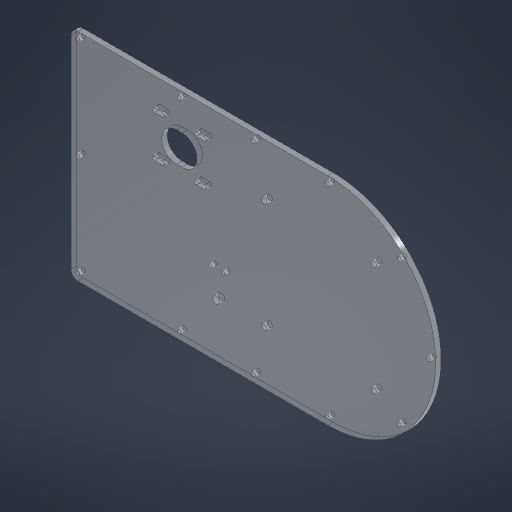
# Autodesk Inventor part: Base_solida
Saved by Autodesk Inventor 2025.2 (Build 292293000, 293)
## iProperties
Created: 2025-04-27
Part Number: Base_solida
Material: Acrilico
Document SubType Name: Modeling
Designer: Tiago
Density: 1.18 g/cm^3
Appearance: Polycarbonate - Clear
Mass: 159.889 g
Surface Area: 836.081 cm^2
Volume: 159.889 cm^3
Author: Tiago
Autodesk Inventor part; units mm, degrees
ref_plane "YZ Plane" through (0, 0, 0) normal (1, 0, 0) x (0, 1, 0)
ref_plane "XZ Plane" through (0, 0, 0) normal (0, 1, 0) x (-1, 0, 0)
ref_plane "XY Plane" through (0, 0, 0) normal (0, 0, 1) x (1, 0, 0)
sketch "Sketch1" plane through (0, 0, 0) normal (0, 0, 1) x (1, 0, 0)
  line L0 (-150, -80) -> (40, -80)
  line L1 (40, 80) -> (-150, 80)
  line L2 (-150, 80) -> (-150, -80)
  line L3 (-150, 0) -> (-107, 0) construction
  line L4 (-107, 0) -> (33.79, 0) construction
  line L5 (33.79, -40.6) -> (33.79, 40.6) construction
  line L6 (-6.81, 0) -> (74.39, 0) construction
  line L7 (33.79, 40.6) -> (74.39, 40.6) construction
  line L8 (74.39, 40.6) -> (74.39, 0) construction
  circle A0 centre (74.39, 40.6) radius 2
  circle A1 centre (74.39, -40.6) radius 2
  circle A2 centre (-6.81, 40.6) radius 2
  circle A3 centre (-6.81, -40.6) radius 2
  line L9 (33.79, 0) -> (33.79, 47) construction
  line L10 (33.79, 0) -> (33.79, -47) construction
  line L11 (150, 0) -> (120, 0) construction
  line L12 (120, 0) -> (120, 0)
  arc A4 (40, -80) -> (120, 0) centre (40, 0) ccw
  arc A5 (120, 0) -> (40, 80) centre (40, 0) ccw
  line L13 (120, 0) -> (115, 0) construction
  circle A6 centre (115, 0) radius 1.5
  line L14 (40, 0) -> (96.5685, 56.5685) construction
  line L15 (96.5685, -56.5685) -> (93.033, -53.033) construction
  circle A7 centre (93.033, -53.033) radius 1.5
  line L16 (40, -80) -> (40, -75) construction
  circle A8 centre (40, -75) radius 1.5
  line L17 (40, -75) -> (-15, -75) construction
  line L18 (-15, -75) -> (-70, -75) construction
  line L19 (-150, -75) -> (-145, -75) construction
  circle A9 centre (-15, -75) radius 1.5
  circle A10 centre (-70, -75) radius 1.5
  circle A11 centre (-145, -75) radius 1.5
  circle A12 centre (-145, 0) radius 1.5
  circle A13 centre (93.033, 53.033) radius 1.5
  circle A14 centre (40, 75) radius 1.5
  circle A15 centre (-15, 75) radius 1.5
  circle A16 centre (-70, 75) radius 1.5
  circle A17 centre (-145, 75) radius 1.5
  line L20 (-145, -80) -> (-145, -75) construction
  line L21 (-150, 0) -> (-145, 0) construction
  line L22 (-71.7142, 42.5) -> (-67.7142, 42.5) construction
  line L23 (33.79, 0) -> (31.29, 0) construction
  line L24 (33.79, 0) -> (45.79, 0) construction
  line L25 (45.79, 0) -> (45.79, 58) construction
  circle A18 centre (45.79, 58) radius 1.1
  circle A19 centre (45.79, 65) radius 1.1
  arc A20 (-82.2142, 56.5) -> (-82.2142, 59.5) centre (-82.2142, 58) ccw
  line L26 (-82.2142, 56.5) -> (-88.2142, 56.5)
  line L27 (-82.2142, 59.5) -> (-88.2142, 59.5)
  arc A21 (-88.2142, 59.5) -> (-88.2142, 56.5) centre (-88.2142, 58) ccw
  arc A22 (-57.2142, 59.5) -> (-57.2142, 56.5) centre (-57.2142, 58) ccw
  line L28 (-57.2142, 56.5) -> (-51.2142, 56.5)
  line L29 (-57.2142, 59.5) -> (-51.2142, 59.5)
  arc A23 (-51.2142, 56.5) -> (-51.2142, 59.5) centre (-51.2142, 58) ccw
  arc A24 (-82.2142, 25.5) -> (-82.2142, 28.5) centre (-82.2142, 27) ccw
  line L30 (-82.2142, 28.5) -> (-88.2142, 28.5)
  line L31 (-82.2142, 25.5) -> (-88.2142, 25.5)
  arc A25 (-88.2142, 28.5) -> (-88.2142, 25.5) centre (-88.2142, 27) ccw
  line L32 (-57.2142, 28.5) -> (-51.2142, 28.5)
  arc A26 (-51.2142, 25.5) -> (-51.2142, 28.5) centre (-51.2142, 27) ccw
  line L33 (-57.2142, 25.5) -> (-51.2142, 25.5)
  arc A27 (-57.2142, 28.5) -> (-57.2142, 25.5) centre (-57.2142, 27) ccw
  arc A28 (-71.7142, 53.5) -> (-71.7142, 31.5) centre (-71.7142, 42.5) ccw
  arc A29 (-67.7142, 31.5) -> (-67.7142, 53.5) centre (-67.7142, 42.5) ccw
  line L34 (-67.7142, 53.5) -> (-71.7142, 53.5)
  line L35 (-67.7142, 31.5) -> (-71.7142, 31.5)
  circle A30 centre (-37.21, -21) radius 1.25
  circle A31 centre (-46.71, -21) radius 1.25
  line L36 (33.79, 0) -> (-69.7142, 42.5) construction
  circle A32 centre (-42.71, -41) radius 2.5
  point P0 (0, 0)
  point P1 (120, -80)
  point P2 (120, 0)
  point P3 (-69.7142, 31.5)
  point P4 (-69.7142, 53.5)
  point P5 (-85.2142, 27)
  point P6 (-54.2142, 27)
  point P7 (-54.2142, 58)
  point P8 (-85.2142, 58)
  point P9 (-54.2142, 25.5)
  point P10 (-58.7142, 58)
  point P11 (-49.7142, 58)
  point P12 (-58.7142, 27)
  point P13 (-49.7142, 27)
  point P14 (-89.7142, 27)
  point P15 (-85.2142, 28.5)
  point P16 (-85.2142, 25.5)
  point P17 (-80.7142, 27)
  point P18 (-89.7142, 58)
  point P19 (-80.7142, 58)
  point P20 (-85.2142, 59.5)
  point P21 (-54.2142, 59.5)
  point P22 (-54.2142, 56.5)
  point P23 (-40.21, -41)
  dimension "d146" = 5
  dimension "d4" = 43
  dimension "d6" = 140.79
  dimension "L_furos" = 81.2
  dimension "d9" = 81.2
  dimension "d11" = 4
  dimension "d30" = 47
  dimension "d47" = 30
  dimension "d49" = 80
  dimension "LF" = 5
  dimension "Furos" = 3
  dimension "d52" = 45
  dimension "d53" = 5
  dimension "d55" = 3
  dimension "d56" = 5
  dimension "d57" = 3
  dimension "d58" = 55
  dimension "d59" = 55
  dimension "d60" = 5
  dimension "d61" = 3
  dimension "d62" = 3
  dimension "d63" = 3
  dimension "d64" = 3
  dimension "d65" = 5
  dimension "d66" = 5
  dimension "d67" = 33.79
  dimension "d68" = 4
  dimension "d72" = 2.5
  dimension "d77" = 12
  dimension "d84" = 3
  dimension "d85" = 1.5
  dimension "d88" = 11
  dimension "d90" = 58
  dimension "d91" = 7
  dimension "d92" = 2.2
  dimension "d93" = 2.2
  dimension "d94" = 80
  dimension "d95" = 80
  dimension "d96" = 40
  dimension "d97" = 150
  dimension "d98" = 2.5
  dimension "d99" = 2.5
  dimension "d102" = 71
  dimension "d103" = 21
  dimension "d115" = 11
  dimension "FF" = 1.5
  dimension "d121" = 1.5
  dimension "d122" = 1.5
  dimension "d124" = 3
  dimension "d125" = 1.5
  dimension "d126" = 1.5
  dimension "d127" = 1.5
  dimension "d128" = 1.5
  dimension "d129" = 15.5
  dimension "d130" = 15.5
  dimension "d131" = 15.5
  dimension "d132" = 15.5
  dimension "d133" = 6
  dimension "DLF" = 6
  dimension "d135" = 6
  dimension "d136" = 6
  dimension "d138" = 42.5
  dimension "d139" = 15.5
  dimension "d140" = 103.5042
  dimension "d141" = 111.89
  constraints: 74 end point, 34 point on circle, 32 centre point, 26 horizontal alignment, 24 tangent, 23 vertical alignment, 21 coincident, 12 midpoint, 12 symmetric about line, 9 horizontal, 6 point on line, 5 equal radius, 5 perpendicular, 3 vertical, 1 parallel, 10 other
  measures "d4" distance of L3.start L3.end
  measures "d6" distance of L4.start L4.end
  measures "L_furos" distance of L5.start L5.end
  measures "d9" distance of L6.start L6.end
  measures "d11" diameter of A0
  measures "d30" distance of L9.start L9.end
  measures "d47" distance of L11.start L11.end
  measures "d49" radius of A4
  measures "LF" distance of L12.end L13.end
  measures "Furos" diameter of A6
  measures "d52" angle of L6 L14
  measures "d53" distance of L15.start L15.end
  measures "d55" diameter of A7
  measures "d56" distance of L0.end L16.end
  measures "d57" diameter of A8
  measures "d58" distance of L17.start L17.end
  measures "d59" distance of L17.end L18.end
  measures "d60" distance of L19.end L19.start
  measures "d61" diameter of A9
  measures "d62" diameter of A10
  measures "d63" diameter of A11
  measures "d64" diameter of A12
  measures "d65" distance of L20.start L19.end
  measures "d66" distance of L3.start L21.end
  measures "d67" distance of L4.end point (0, 0)
  measures "d68" distance of L22.start L22.end
  measures "d72" distance of L23.start L23.end
  measures "d77" distance of L23.start L24.end
  measures "d84" diameter of A20
  measures "d85" radius of A21
  measures "d88" radius of A29
  measures "d90" distance of L24.end L25.end
  measures "d91" distance of A19.centre L25.end
  measures "d92" diameter of A18
  measures "d93" diameter of A19
  measures "d94" distance from line of point (0, 0) L1
  measures "d95" distance from line of L0 point (0, 0)
  measures "d96" distance of A4.centre point (0, 0)
  measures "d97" distance from line of point (0, 0) L2
  measures "d98" diameter of A30
  measures "d99" diameter of A31
  measures "d102" horizontal distance of point (33.79, 0) A30.centre
  measures "d103" distance from line of L4 A30.centre
  measures "d115" distance of point (-69.714, 31.5) L36.end
  measures "FF" radius of A22
  measures "d121" radius of A27
  measures "d122" radius of A24
  measures "d124" distance between parallel lines of L32 L33
  measures "d125" distance of point (-54.214, 25.5) point (-54.214, 27)
  measures "d126" distance from line of L29 point (-54.214, 58)
  measures "d127" distance from line of point (-85.214, 27) L31
  measures "d128" distance from line of point (-85.214, 58) L26
  measures "d129" horizontal distance of point (-69.714, 42.5) point (-54.214, 27)
  measures "d130" horizontal distance of point (-54.214, 58) L36.end
  measures "d131" horizontal distance of point (-54.214, 58) L36.end
  measures "d132" horizontal distance of point (-54.214, 27) L36.end
  measures "d133" distance of A25.centre A24.centre
  measures "DLF" distance of A26.centre A27.centre
  measures "d135" distance of L26.start L26.end
  measures "d136" distance of L28.end L28.start
  measures "d138" distance from line of L4 L36.end
  measures "d139" horizontal distance of point (-85.214, 27) L36.end
  measures "d140" horizontal distance of L4.end L36.end
  measures "d141" distance of L23.start L36.end
extrude "Extrusion1" add sketch "Sketch1" along normal blind 4 contours L2 L1 A5 A4 L0 | A18 | A19 | A30 | A31 | A32
extrude "Extrusion5" cut sketch "Sketch1" along normal up to surface (4 mm away) contours A30 | A31 | A32
fillet "Fillet1" radius 5 2 edges at (-150, -80, 2) (-150, 80, 2)
equation "\"d9\" = L_furos"
equation "\"d53\" = LF"
equation "\"d55\" = Furos"
equation "\"d56\" = LF"
equation "\"d57\" = Furos"
equation "\"d60\" = LF"
equation "\"d61\" = Furos"
equation "\"d62\" = Furos"
equation "\"d63\" = Furos"
equation "\"d64\" = Furos"
equation "\"d65\" = LF"
equation "\"d66\" = LF"
body "Solid1"
